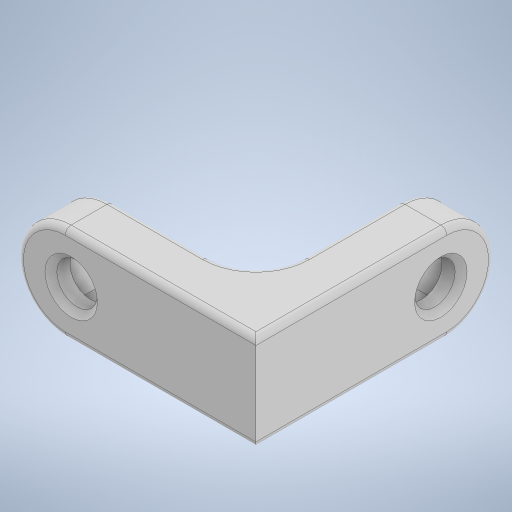
# Autodesk Inventor part: BoxBracket
Saved by Autodesk Inventor 2023 (Build 270158000, 158)
## iProperties
Created: 2023-11-15
Part Number: BoxBracket
Material: Generic
Document SubType Name: Modeling
Designer: Eric
Density: 1 g/cm^3
Appearance: Default
Author: Eric
Autodesk Inventor part; units mm, degrees
ref_plane "YZ Plane" through (0, 0, 0) normal (1, 0, 0) x (0, 1, 0)
ref_plane "XZ Plane" through (0, 0, 0) normal (0, 1, 0) x (-1, 0, 0)
ref_plane "XY Plane" through (0, 0, 0) normal (0, 0, 1) x (1, 0, 0)
sketch "Sketch1" plane through (0, 0, 0) normal (1, 0, 0) x (0, 1, 0)
  line L0 (0, 0) -> (8, 0)
  line L1 (8, 0) -> (8, -20)
  line L2 (8, -20) -> (0, -20)
  line L3 (0, -20) -> (0, 0)
  dimension "d0" = 8
  dimension "d1" = 20
  constraints: 8 end point, 2 parallel, 1 horizontal, 1 perpendicular
  measures "d0" distance of L1.end L2.end
  measures "d1" distance of L0.end L1.end
extrude "Extrusion1" add sketch "Sketch1" against normal blind 4
sketch "Sketch2" plane through (0, 0, 0) normal (0, 0, 1) x (1, 0, 0)
  line L0 (0, 0) -> (-4, 0) projected
  line L1 (0, 0) -> (-20, 0)
  line L2 (-20, 0) -> (-20, 8)
  line L3 (-20, 8) -> (0, 8)
  line L4 (0, 8) -> (0, 0)
  line L5 (0, 8) -> (0, 0) projected
  dimension "d4" = 20
  constraints: 8 end point, 2 parallel, 1 collinear, 1 horizontal, 1 perpendicular
  measures "d4" distance of L2.end L3.end
extrude "Extrusion2" add sketch "Sketch2" against normal blind 4
sketch "Sketch3" plane through (-4, 0, 0) normal (-1, 0, 0) x (0, 0, 1)
  line L0 (-13.9123, 1.25) -> (-17.0877, 1.25)
  line L1 (-17.0877, 1.25) -> (-18.6754, 4)
  line L2 (-18.6754, 4) -> (-17.0877, 6.75)
  line L3 (-17.0877, 6.75) -> (-13.9123, 6.75)
  line L4 (-13.9123, 6.75) -> (-12.3246, 4)
  line L5 (-12.3246, 4) -> (-13.9123, 1.25)
  line L6 (-20, 8) -> (-20, 0) projected
  point P0 (0, 0)
  point P1 (-15.5, 4)
  point P2 (-20, 4)
  dimension "d7" = 5.5
  dimension "d8" = 4.5
  constraints: 12 end point, 1 horizontal, 1 horizontal alignment, 1 midpoint, 13 other
  measures "d7" distance between parallel lines of L0 L3
  measures "d8" distance from line of L6 point (-15.5, 4)
extrude "Extrusion3" cut sketch "Sketch3" against normal blind 2.4
sketch "Sketch4" plane through (-1.6, 0, 0) normal (-1, 0, 0) x (0, 0, 1)
  line L0 (-13.9123, 6.75) -> (-12.3246, 4) projected
  line L1 (-17.0877, 6.75) -> (-13.9123, 6.75) projected
  line L2 (-18.6754, 4) -> (-17.0877, 6.75) projected
  line L3 (-17.0877, 1.25) -> (-18.6754, 4) projected
  line L4 (-13.9123, 1.25) -> (-17.0877, 1.25) projected
  line L5 (-12.3246, 4) -> (-13.9123, 1.25) projected
  circle A0 centre (-15.5, 4) radius 1.7
  point P0 (0, 0)
  dimension "d11" = 3.4
  constraints: 1 centre point, 1 coincident
  measures "d11" diameter of A0
extrude "Extrusion4" cut sketch "Sketch4" against normal up to surface (1.6 mm away) contours A0
sketch "Sketch5" plane through (0, 0, -4) normal (0, 0, -1) x (-1, 0, 0)
  line L0 (17.0877, 1.25) -> (13.9123, 1.25)
  line L1 (13.9123, 1.25) -> (12.3246, 4)
  line L2 (12.3246, 4) -> (13.9123, 6.75)
  line L3 (13.9123, 6.75) -> (17.0877, 6.75)
  line L4 (17.0877, 6.75) -> (18.6754, 4)
  line L5 (18.6754, 4) -> (17.0877, 1.25)
  line L6 (20, 0) -> (20, 8) projected
  point P0 (0, 0)
  point P1 (15.5, 4)
  point P2 (20, 4)
  dimension "d14" = 5.5
  dimension "d15" = 4.5
  constraints: 12 end point, 1 horizontal, 1 horizontal alignment, 1 midpoint, 13 other
  measures "d14" distance between parallel lines of L3 L0
  measures "d15" distance from line of L6 point (15.5, 4)
extrude "Extrusion5" cut sketch "Sketch5" against normal blind 2.4
sketch "Sketch6" plane through (0, 0, -1.6) normal (0, 0, -1) x (-1, 0, 0)
  circle A0 centre (15.5, 4) radius 1.7
  point P0 (0, 0)
  dimension "d18" = 3.4
  constraints: 1 centre point, 1 coincident
  measures "d18" diameter of A0
extrude "Extrusion6" cut sketch "Sketch6" against normal up to surface (1.6 mm away)
fillet "Fillet1" radius 4 4 edges at (-2, 8, -20) (-2, 0, -20) (-20, 8, -2) (-20, 0, -2)
fillet "Fillet2" radius 4 1 edges at (-4, 4, -4)
fillet "Fillet3" radius 0.5 22 edges at (-4, 8, -12) (-4, 6.8285, -18.8285) (-4, 4, -20) (-4, 1.1715, -18.8285) (-4, 0, -12) (-5.1716, 0, -5.1716) (-12, 0, -4) (-18.8285, 6.8285, -4) (-20, 4, -4) (-18.8285, 1.1715, -4) (-12, 8, -4) (-5.1716, 8, -5.1716) (0, 1.1715, -18.8285) (0, 6.8285, -18.8285) (0, 4, -20) (0, 0, -8) (0, 8, -8) (-18.8285, 1.1715, 0) (-18.8285, 6.8285, 0) (-20, 4, 0) (-8, 0, 0) (-8, 8, 0)
chamfer "Chamfer1" distance 0.5 angle 45 2 edges at (0, 4, -17.2) (-13.8, 4, 0)
body "Solid1"
